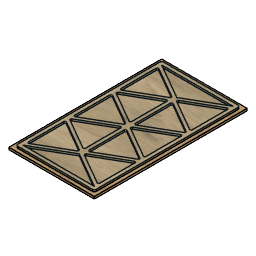
Game Board (Autodesk Fusion 360 design; units mm, degrees)
Autodesk Fusion 360 part; units mm, degrees
note: some values were not read from the file. Set by a fixed rule: which sketch regions a step uses.
sketch "Sketch1" plane through (0, 0, 0) normal (0, 1, 0) x (1, 0, 0) in component "Divider"
  line L0 (0, 0) -> (127.3337, 73.5162)
  line L1 (5.715, 15.9996) -> (115.2687, 79.2504)
  line L2 (115.2687, 85.8496) -> (5.715, 149.1004)
  line L3 (0, 145.8009) -> (0, 19.2991)
  line L4 (127.3337, 73.5162) -> (127.3337, 421.7835) construction
  line L5 (115.2687, 98.5496) -> (5.715, 161.8004)
  line L6 (5.715, 168.3996) -> (115.2687, 231.6504)
  line L7 (120.9837, 228.3509) -> (120.9837, 101.8491)
  line L8 (115.2687, 244.3504) -> (5.715, 181.0996)
  line L9 (0, 184.3991) -> (0, 310.9009)
  line L10 (5.715, 314.2004) -> (115.2687, 250.9496)
  line L11 (5.715, 326.9004) -> (115.2687, 263.6496)
  line L12 (120.9837, 266.9491) -> (120.9837, 393.4509)
  line L13 (115.2687, 396.7504) -> (5.715, 333.4996)
  line L14 (5.715, 346.1996) -> (115.2687, 409.4504)
  line L15 (115.2687, 416.0496) -> (5.715, 479.3004)
  line L16 (0, 476.0009) -> (0, 349.4991)
  line L17 (127.3337, 421.7835) -> (8.2094, 490.5599)
  line L18 (0, -12.7) -> (-5.08, -12.7)
  line L19 (-12.7, -5.08) -> (-12.7, 0)
  line L20 (-12.7, 495.2996) -> (-12.7, 500.3796)
  line L21 (0, 507.9996) -> (-5.08, 507.9996)
  line L22 (-12.7, 495.2996) -> (-12.7, 0)
  line L23 (127.3337, 421.7835) -> (246.4581, 490.5599)
  line L24 (267.3675, -5.08) -> (267.3675, 0)
  line L25 (267.3675, 495.2996) -> (267.3675, 0)
  line L26 (254.6675, 507.9996) -> (259.7475, 507.9996)
  line L27 (254.6675, -12.7) -> (259.7475, -12.7)
  line L28 (254.6675, 0) -> (127.3337, 73.5162)
  line L29 (267.3675, 495.2996) -> (267.3675, 500.3796)
  line L30 (9.4794, 495.2996) -> (245.1881, 495.2996)
  line L31 (0, 0) -> (254.6675, 0)
  line L32 (0, -12.7) -> (254.6675, -12.7)
  line L33 (0, 507.9996) -> (254.6675, 507.9996)
  arc A0 (0, 19.2991) -> (5.715, 15.9996) centre (3.81, 19.2991) ccw
  arc A1 (5.715, 149.1004) -> (0, 145.8009) centre (3.81, 145.8009) ccw
  arc A2 (115.2687, 79.2504) -> (115.2687, 85.8496) centre (113.3637, 82.55) ccw
  arc A3 (5.715, 168.3996) -> (5.715, 161.8004) centre (7.62, 165.1) ccw
  arc A4 (115.2687, 98.5496) -> (120.9837, 101.8491) centre (117.1737, 101.8491) ccw
  arc A5 (120.9837, 228.3509) -> (115.2687, 231.6504) centre (117.1737, 228.3509) ccw
  arc A6 (0, 184.3991) -> (5.715, 181.0996) centre (3.81, 184.3991) ccw
  arc A7 (115.2687, 244.3504) -> (115.2687, 250.9496) centre (113.3637, 247.65) ccw
  arc A8 (5.715, 314.2004) -> (0, 310.9009) centre (3.81, 310.9009) ccw
  arc A9 (5.715, 333.4996) -> (5.715, 326.9004) centre (7.62, 330.2) ccw
  arc A10 (115.2687, 263.6496) -> (120.9837, 266.9491) centre (117.1737, 266.9491) ccw
  arc A11 (120.9837, 393.4509) -> (115.2687, 396.7504) centre (117.1737, 393.4509) ccw
  arc A12 (115.2687, 409.4504) -> (115.2687, 416.0496) centre (113.3637, 412.75) ccw
  arc A13 (0, 349.4991) -> (5.715, 346.1996) centre (3.81, 349.4991) ccw
  arc A14 (5.715, 479.3004) -> (0, 476.0009) centre (3.81, 476.0009) ccw
  line L34 (254.6675, 145.8009) -> (254.6675, 19.2991)
  line L35 (248.9525, 15.9996) -> (139.3987, 79.2504)
  line L36 (139.3987, 85.8496) -> (248.9525, 149.1004)
  arc A15 (254.6675, 145.8009) -> (248.9525, 149.1004) centre (250.8575, 145.8009) ccw
  arc A16 (139.3987, 85.8496) -> (139.3987, 79.2504) centre (141.3037, 82.55) ccw
  arc A17 (248.9525, 15.9996) -> (254.6675, 19.2991) centre (250.8575, 19.2991) ccw
  line L37 (139.3987, 98.5496) -> (248.9525, 161.8004)
  line L38 (248.9525, 168.3996) -> (139.3987, 231.6504)
  arc A18 (248.9525, 161.8004) -> (248.9525, 168.3996) centre (247.0475, 165.1) ccw
  arc A19 (139.3987, 231.6504) -> (133.6837, 228.3509) centre (137.4937, 228.3509) ccw
  line L39 (133.6837, 228.3509) -> (133.6837, 101.8491)
  arc A20 (133.6837, 101.8491) -> (139.3987, 98.5496) centre (137.4937, 101.8491) ccw
  line L40 (139.3987, 244.3504) -> (248.9525, 181.0996)
  arc A21 (248.9525, 181.0996) -> (254.6675, 184.3991) centre (250.8575, 184.3991) ccw
  line L41 (254.6675, 184.3991) -> (254.6675, 310.9009)
  arc A22 (254.6675, 310.9009) -> (248.9525, 314.2004) centre (250.8575, 310.9009) ccw
  line L42 (248.9525, 314.2004) -> (139.3987, 250.9496)
  arc A23 (139.3987, 250.9496) -> (139.3987, 244.3504) centre (141.3037, 247.65) ccw
  arc A24 (133.6837, 266.9491) -> (139.3987, 263.6496) centre (137.4937, 266.9491) ccw
  line L43 (248.9525, 326.9004) -> (139.3987, 263.6496)
  arc A25 (248.9525, 326.9004) -> (248.9525, 333.4996) centre (247.0475, 330.2) ccw
  line L44 (139.3987, 396.7504) -> (248.9525, 333.4996)
  line L45 (133.6837, 266.9491) -> (133.6837, 393.4509)
  arc A26 (139.3987, 396.7504) -> (133.6837, 393.4509) centre (137.4937, 393.4509) ccw
  arc A27 (139.3987, 416.0496) -> (139.3987, 409.4504) centre (141.3037, 412.75) ccw
  line L46 (248.9525, 346.1996) -> (139.3987, 409.4504)
  line L47 (139.3987, 416.0496) -> (248.9525, 479.3004)
  arc A28 (248.9525, 346.1996) -> (254.6675, 349.4991) centre (250.8575, 349.4991) ccw
  line L48 (254.6675, 476.0009) -> (254.6675, 349.4991)
  arc A29 (254.6675, 476.0009) -> (248.9525, 479.3004) centre (250.8575, 476.0009) ccw
  line L49 (-25.4, -25.4) -> (280.0675, -25.4)
  line L50 (280.0675, -25.4) -> (280.0675, 520.6996)
  line L51 (280.0675, 520.6996) -> (-25.4, 520.6996)
  line L52 (-25.4, 520.6996) -> (-25.4, -25.4)
  arc A30 (-12.7, -5.08) -> (-5.08, -12.7) centre (-5.08, -5.08) ccw
  arc A31 (-5.08, 507.9996) -> (-12.7, 500.3796) centre (-5.08, 500.3796) ccw
  arc A32 (267.3675, 500.3796) -> (259.7475, 507.9996) centre (259.7475, 500.3796) ccw
  arc A33 (259.7475, -12.7) -> (267.3675, -5.08) centre (259.7475, -5.08) ccw
  line L53 (246.4581, 490.5599) -> (254.6675, 495.2996)
  line L54 (254.6675, 495.2996) -> (245.1881, 495.2996)
  line L55 (8.2094, 490.5599) -> (0, 495.2996)
  line L56 (0, 495.2996) -> (9.4794, 495.2996)
  point P0 (0, 12.7)
  point P1 (120.9837, 82.55)
  point P2 (0, 152.4)
  point P3 (120.9837, 95.25)
  point P4 (0, 165.1)
  point P5 (120.9837, 234.95)
  point P6 (120.9837, 247.65)
  point P7 (0, 177.8)
  point P8 (0, 317.5)
  point P9 (0, 330.2)
  point P10 (120.9837, 260.35)
  point P11 (120.9837, 400.05)
  point P12 (0, 342.9)
  point P13 (120.9837, 412.75)
  point P14 (0, 482.6)
  point P15 (0, 495.2996)
  point P16 (-12.7, -12.7)
  point P17 (267.3675, 507.9996)
  point P18 (254.6675, 0)
  dimension "d7" = 139.7
  dimension "d8" = 139.7
  dimension "d9" = 60
  dimension "d10" = 12.7
  dimension "d12" = 127.3337
  dimension "d14" = 139.7
  dimension "d15" = 139.7
  dimension "d16" = 12.7
  dimension "d17" = 12.7
  dimension "d19" = 139.7
  dimension "d20" = 139.7
  dimension "d21" = 139.7
  dimension "d22" = 6.35
  dimension "d23" = 12.7
  dimension "d24" = 12.7
  dimension "d26" = 139.7
  dimension "d27" = 139.7
  dimension "d28" = 6.35
  dimension "d29" = 12.7
  dimension "d30" = 6.35
  dimension "d31" = 139.7
  dimension "d32" = 139.7
  dimension "d34" = 10.9982
  dimension "d35" = 12.7
  dimension "d36" = 12.7
  dimension "d38" = 12.7
  dimension "d39" = 12.7
  dimension "d43" = 12.7
  dimension "d44" = 12.7
  dimension "d45" = 12.7
  dimension "d46" = 12.7
  dimension "d48" = 254.6675
  dimension "d201" = 3.81
  dimension "d202" = 3.81
  dimension "d203" = 3.81
  dimension "d204" = 3.81
  dimension "d205" = 3.81
  dimension "d206" = 3.81
  dimension "d207" = 3.81
  dimension "d208" = 3.81
  dimension "d209" = 3.81
  dimension "d210" = 3.81
  dimension "d211" = 3.81
  dimension "d212" = 3.81
  dimension "d213" = 3.81
  dimension "d214" = 3.81
  dimension "d215" = 3.81
  dimension "d216" = 12.7
  dimension "d217" = 6.35
  dimension "d218" = 12.7
  dimension "d219" = 12.7
  dimension "d220" = 12.7
  dimension "d221" = 12.7
  dimension "d230" = 7.62
  dimension "d231" = 7.62
  dimension "d232" = 7.62
  dimension "d233" = 7.62
  constraint coincident L0.start L31.start
  constraint vertical L3
  constraint vertical L0.start P0
  constraint parallel L0 L1
  constraint vertical L4
  constraint parallel L6 L8
  constraint vertical L9
  constraint parallel L10 L11
  constraint parallel L9 L12
  constraint parallel L13 L14
  constraint vertical L16
  constraint parallel L15 L17
  constraint vertical P14 P15
  constraint perpendicular L20 L21
  constraint perpendicular L18 L22
  constraint symmetric L0.start L4 P18
  constraint symmetric L0.end L4 L28.end
  constraint symmetric L4 L17.start L23.start
  constraint symmetric L4 L19.end L24.end
  constraint symmetric L4 L18.start L27.start
  constraint symmetric L4 L21.start L26.start
  constraint symmetric L4 L20.start L25.start
  constraint coincident P18 L28.start
  constraint parallel L26 L33
  constraint coincident P0 L1
  constraint tangent L1 A0
  constraint tangent L3 A0
  constraint coincident P2 L3
  constraint tangent L2 A1
  constraint tangent L3 A1
  constraint coincident P1 L2
  constraint coincident P1 L1
  constraint tangent L2 A2
  constraint tangent L1 A2
  constraint coincident P4 L5
  constraint tangent L6 A3
  constraint tangent L5 A3
  constraint coincident P3 L5
  constraint coincident P3 L7
  constraint tangent L5 A4
  constraint tangent L7 A4
  constraint coincident P5 L6
  constraint coincident P5 L7
  constraint tangent L6 A5
  constraint tangent L7 A5
  constraint coincident P7 L8
  constraint coincident P7 L9
  constraint tangent L8 A6
  constraint tangent L9 A6
  constraint coincident P6 L10
  constraint coincident P6 L8
  constraint tangent L10 A7
  constraint tangent L8 A7
  constraint coincident P8 L9
  constraint coincident P8 L10
  constraint tangent L9 A8
  constraint tangent L10 A8
  constraint coincident P9 L13
  constraint coincident P9 L11
  constraint tangent L13 A9
  constraint tangent L11 A9
  constraint coincident P10 L11
  constraint coincident P10 L12
  constraint tangent L11 A10
  constraint tangent L12 A10
  constraint coincident P11 L13
  constraint coincident P11 L12
  constraint tangent L13 A11
  constraint tangent L12 A11
  constraint coincident P13 L15
  constraint coincident P13 L14
  constraint tangent L15 A12
  constraint tangent L14 A12
  constraint coincident P12 L16
  constraint coincident P12 L14
  constraint tangent L16 A13
  constraint tangent L14 A13
  constraint coincident P14 L16
  constraint coincident P14 L15
  constraint tangent L16 A14
  constraint tangent L15 A14
  constraint symmetric L4 L1.start L35.start
  constraint symmetric L4 L3.end L34.end
  constraint symmetric L4 A0 A17
  constraint symmetric L4 L2.end L36.end
  constraint symmetric L4 L3.start L34.start
  constraint symmetric L4 A1 A15
  constraint symmetric L4 L2.start L36.start
  constraint symmetric L4 L1.end L35.end
  constraint symmetric L4 A2 A16
  constraint symmetric L4 L6.start L38.start
  constraint symmetric L4 L5.end L37.end
  constraint symmetric L4 A3 A18
  constraint symmetric L4 L5.start L37.start
  constraint symmetric L4 L7.end L39.end
  constraint symmetric L4 A4 A20
  constraint symmetric L4 L6.end L38.end
  constraint symmetric L4 L7.start A19.end
  constraint symmetric L4 A5 A19
  constraint symmetric L4 L8.end L40.end
  constraint symmetric L4 L9.start A21.end
  constraint symmetric L4 A6 A21
  constraint symmetric L4 L10.end L42.end
  constraint symmetric L4 L8.start L40.start
  constraint symmetric L4 A7 A23
  constraint symmetric L4 L9.end L41.end
  constraint symmetric L4 L10.start A22.end
  constraint symmetric L4 A8 A22
  constraint symmetric L4 L13.end A25.end
  constraint symmetric L4 L11.start L43.start
  constraint symmetric L4 A9 A25
  constraint symmetric L4 L11.end A24.end
  constraint symmetric L4 L12.start A24.start
  constraint symmetric L4 A10 A24
  constraint symmetric L4 L13.start L44.start
  constraint symmetric L4 L12.end L45.end
  constraint symmetric L4 A11 A26
  constraint symmetric L4 L15.start A27.start
  constraint symmetric L4 L14.end A27.end
  constraint symmetric L4 A12 A27
  constraint symmetric L4 L16.end A28.end
  constraint symmetric L4 L14.start L46.start
  constraint symmetric L4 A13 A28
  constraint symmetric L4 L16.start L48.start
  constraint symmetric L4 L15.end L47.end
  constraint symmetric L4 A14 A29
  constraint horizontal L49
  constraint vertical L50
  constraint horizontal L51
  constraint vertical L52
  constraint coincident P16 L18
  constraint coincident P16 L19
  constraint tangent L18 A30
  constraint tangent L19 A30
  constraint tangent L20 A31
  constraint tangent L21 A31
  constraint coincident P17 L26
  constraint coincident P17 L29
  constraint tangent L26 A32
  constraint tangent L29 A32
  constraint tangent L24 A33
  constraint tangent L27 A33
  constraint coincident P15 L30
  constraint coincident P15 L17
  constraint parallel L23 L47
  constraint parallel L23 L53
  constraint parallel L30 L54
  constraint coincident P15 L55.end
  measures "d7" distance of P0 P1
  measures "d8" distance of P1 P2
  measures "d9" angle of L2 L3
  measures "d10" vertical distance of L0.start P0
  measures "d12" horizontal distance of L0.start L0.end
  measures "d14" distance of P4 P5
  measures "d15" vertical distance of P3 P5
  measures "d16" vertical distance of P1 P3
  measures "d17" distance of P2 P4
  measures "d19" distance of P3 P4
  measures "d20" distance of P6 P7
  measures "d21" distance of P7 P8
  measures "d22" distance of L4 P6
  measures "d23" distance of P4 P7
  measures "d24" distance of P8 P9
  measures "d26" distance of P9 P11
  measures "d27" distance of P9 P10
  measures "d28" distance of L4 P11
  measures "d29" distance of P9 P12
  measures "d30" distance of L4 P13
  measures "d31" distance of P12 P14
  measures "d32" distance of P13 P14
  measures "d34" distance of L15 L17
  measures "d35" distance of L0.start L19.end
  measures "d36" distance of L0.start L18.start
  measures "d38" distance of P15 L21.start
  measures "d39" distance of P15 L20.start
  measures "d43" distance of P17 L25.start
  measures "d44" distance of P17 L26.start
  measures "d45" distance of L19.end P16
  measures "d46" distance of L18.start P16
  measures "d48" distance of L18.start L27.start
  measures "d201" radius of A0
  measures "d202" radius of A1
  measures "d203" radius of A2
  measures "d204" radius of A3
  measures "d205" radius of A4
  measures "d206" radius of A5
  measures "d207" radius of A6
  measures "d208" radius of A7
  measures "d209" radius of A8
  measures "d210" radius of A9
  measures "d211" radius of A10
  measures "d212" radius of A11
  measures "d213" radius of A12
  measures "d214" radius of A13
  measures "d215" radius of A14
  measures "d216" distance of L25 L34
  measures "d217" distance of L4 L39
  measures "d218" distance of L33 L51
  measures "d219" distance of L32 L49
  measures "d220" distance of L25 L50
  measures "d221" distance of L20 L52
  measures "d230" radius of A30
  measures "d231" radius of A31
  measures "d232" radius of A32
  measures "d233" radius of A33
extrude "Extrude1" add sketch "Sketch1" along normal blind 11.1252 and the other way blind -7.9502 contours L18 L19 L20 L21 L22 L24 L25 L26 L27 L29 L32 L33 A30 A31 A32 A33 in component "Divider"
extrude "Extrude27" add sketch "Sketch1" along normal blind 7.9502 contours L0 L28 L31 | L1 L2 L3 A0 A1 A2 | L5 L6 L7 A3 A4 A5 | L8 L9 L10 A6 A7 A8 | L11 L12 L13 A9 A10 A11 | L14 L15 L16 A12 A13 A14 | L17 L23 L30 L53 L54 L55 L56 | L18 L19 L20 L21 L22 L24 L25 L26 L27 L29 L32 L33 A30 A31 A32 A33 | L34 L35 L36 A15 A16 A17 | L37 L38 A18 A19 L39 A20 | L40 A21 L41 A22 L42 A23 | A24 L43 A25 L44 L45 A26 | A27 L46 L47 A28 L48 A29 | L49 L50 L51 L52 in component "Divider"
extrude "Extrude28" add sketch "Sketch1" along normal blind 14.3002 and the other way blind -11.1252 contours L18 L19 L20 L21 L22 L24 L25 L26 L27 L29 L32 L33 A30 A31 A32 A33 in component "Divider"
sketch "Sketch11" plane through (0, 14.3002, 0) normal (0, 1, 0) x (-1, 0, 0)
  line L0 (-254.6675, 0) -> (0, 0)
  line L1 (0, 0) -> (-127.3337, -73.5162)
  line L2 (-127.3337, -73.5162) -> (-254.6675, 0)
  line L3 (-254.6675, -495.2996) -> (-127.3337, -421.7835)
  line L4 (-127.3337, -421.7835) -> (0, -495.2996)
  line L5 (0, -495.2996) -> (-254.6675, -495.2996)
  arc A0 (-248.9525, -326.9004) -> (-248.9525, -333.4996) centre (-247.0475, -330.2) ccw
  line L6 (-248.9525, -326.9004) -> (-139.3987, -263.6496)
  arc A1 (-133.6837, -266.9491) -> (-139.3987, -263.6496) centre (-137.4937, -266.9491) ccw
  line L7 (-133.6837, -266.9491) -> (-133.6837, -393.4509)
  arc A2 (-139.3987, -396.7504) -> (-133.6837, -393.4509) centre (-137.4937, -393.4509) ccw
  line L8 (-139.3987, -396.7504) -> (-248.9525, -333.4996)
  arc A3 (-115.2687, -98.5496) -> (-120.9837, -101.8491) centre (-117.1737, -101.8491) ccw
  line L9 (-115.2687, -98.5496) -> (-5.715, -161.8004)
  arc A4 (-5.715, -168.3996) -> (-5.715, -161.8004) centre (-7.62, -165.1) ccw
  line L10 (-5.715, -168.3996) -> (-115.2687, -231.6504)
  arc A5 (-120.9837, -228.3509) -> (-115.2687, -231.6504) centre (-117.1737, -228.3509) ccw
  line L11 (-120.9837, -228.3509) -> (-120.9837, -101.8491)
  arc A6 (-115.2687, -244.3504) -> (-115.2687, -250.9496) centre (-113.3637, -247.65) ccw
  line L12 (-115.2687, -244.3504) -> (-5.715, -181.0996)
  arc A7 (0, -184.3991) -> (-5.715, -181.0996) centre (-3.81, -184.3991) ccw
  line L13 (0, -184.3991) -> (0, -310.9009)
  arc A8 (-5.715, -314.2004) -> (0, -310.9009) centre (-3.81, -310.9009) ccw
  line L14 (-5.715, -314.2004) -> (-115.2687, -250.9496)
  arc A9 (-133.6837, -101.8491) -> (-139.3987, -98.5496) centre (-137.4937, -101.8491) ccw
  line L15 (-133.6837, -101.8491) -> (-133.6837, -228.3509)
  arc A10 (-139.3987, -231.6504) -> (-133.6837, -228.3509) centre (-137.4937, -228.3509) ccw
  line L16 (-139.3987, -231.6504) -> (-248.9525, -168.3996)
  arc A11 (-248.9525, -161.8004) -> (-248.9525, -168.3996) centre (-247.0475, -165.1) ccw
  line L17 (-248.9525, -161.8004) -> (-139.3987, -98.5496)
  arc A12 (-248.9525, -346.1996) -> (-254.6675, -349.4991) centre (-250.8575, -349.4991) ccw
  line L18 (-248.9525, -346.1996) -> (-139.3987, -409.4504)
  arc A13 (-139.3987, -416.0496) -> (-139.3987, -409.4504) centre (-141.3037, -412.75) ccw
  line L19 (-139.3987, -416.0496) -> (-248.9525, -479.3004)
  arc A14 (-254.6675, -476.0009) -> (-248.9525, -479.3004) centre (-250.8575, -476.0009) ccw
  line L20 (-254.6675, -476.0009) -> (-254.6675, -349.4991)
  arc A15 (-115.2687, -79.2504) -> (-115.2687, -85.8496) centre (-113.3637, -82.55) ccw
  line L21 (-115.2687, -79.2504) -> (-5.715, -15.9996)
  arc A16 (0, -19.2991) -> (-5.715, -15.9996) centre (-3.81, -19.2991) ccw
  line L22 (0, -19.2991) -> (0, -145.8009)
  arc A17 (-5.715, -149.1004) -> (0, -145.8009) centre (-3.81, -145.8009) ccw
  line L23 (-5.715, -149.1004) -> (-115.2687, -85.8496)
  arc A18 (-139.3987, -250.9496) -> (-139.3987, -244.3504) centre (-141.3037, -247.65) ccw
  line L24 (-139.3987, -250.9496) -> (-248.9525, -314.2004)
  arc A19 (-254.6675, -310.9009) -> (-248.9525, -314.2004) centre (-250.8575, -310.9009) ccw
  line L25 (-254.6675, -310.9009) -> (-254.6675, -184.3991)
  arc A20 (-248.9525, -181.0996) -> (-254.6675, -184.3991) centre (-250.8575, -184.3991) ccw
  line L26 (-248.9525, -181.0996) -> (-139.3987, -244.3504)
  arc A21 (-139.3987, -85.8496) -> (-139.3987, -79.2504) centre (-141.3037, -82.55) ccw
  line L27 (-139.3987, -85.8496) -> (-248.9525, -149.1004)
  arc A22 (-254.6675, -145.8009) -> (-248.9525, -149.1004) centre (-250.8575, -145.8009) ccw
  line L28 (-254.6675, -145.8009) -> (-254.6675, -19.2991)
  arc A23 (-248.9525, -15.9996) -> (-254.6675, -19.2991) centre (-250.8575, -19.2991) ccw
  line L29 (-248.9525, -15.9996) -> (-139.3987, -79.2504)
  arc A24 (-5.715, -479.3004) -> (0, -476.0009) centre (-3.81, -476.0009) ccw
  line L30 (-5.715, -479.3004) -> (-115.2687, -416.0496)
  arc A25 (-115.2687, -409.4504) -> (-115.2687, -416.0496) centre (-113.3637, -412.75) ccw
  line L31 (-115.2687, -409.4504) -> (-5.715, -346.1996)
  arc A26 (0, -349.4991) -> (-5.715, -346.1996) centre (-3.81, -349.4991) ccw
  line L32 (0, -349.4991) -> (0, -476.0009)
  arc A27 (-120.9837, -393.4509) -> (-115.2687, -396.7504) centre (-117.1737, -393.4509) ccw
  line L33 (-120.9837, -393.4509) -> (-120.9837, -266.9491)
  arc A28 (-115.2687, -263.6496) -> (-120.9837, -266.9491) centre (-117.1737, -266.9491) ccw
  line L34 (-115.2687, -263.6496) -> (-5.715, -326.9004)
  arc A29 (-5.715, -333.4996) -> (-5.715, -326.9004) centre (-7.62, -330.2) ccw
  line L35 (-5.715, -333.4996) -> (-115.2687, -396.7504)
  line L36 (5.08, 12.7) -> (-259.7475, 12.7)
  arc A30 (-259.7475, 12.7) -> (-267.3675, 5.08) centre (-259.7475, 5.08) ccw
  line L37 (-267.3675, 5.08) -> (-267.3675, -500.3796)
  arc A31 (-267.3675, -500.3796) -> (-259.7475, -507.9996) centre (-259.7475, -500.3796) ccw
  line L38 (-259.7475, -507.9996) -> (5.08, -507.9996)
  arc A32 (5.08, -507.9996) -> (12.7, -500.3796) centre (5.08, -500.3796) ccw
  line L39 (12.7, -500.3796) -> (12.7, 5.08)
  arc A33 (12.7, 5.08) -> (5.08, 12.7) centre (5.08, 5.08) ccw
component "Divider" placed x (1, 0, 0) y (0, 1, 0) z (0, 0, 1) at (0, 0, 0)
equation "d12 = 4.7631397208 in + 0.25 in"
equation "d226 = 0.438 in + 0.125 in"
